Autodesk Fusion 360 part; units mm, degrees
(part 3 of 3)
  spline S37 degree 5 poles (-0.7155, 73.9902) (-0.7207, 73.9804) (-0.7312, 73.9608) (-0.7469, 73.9314) (-0.7676, 73.8922) (-0.7933, 73.8432) (-0.8188, 73.7941) (-0.844, 73.7449) (-0.8689, 73.6957) (-0.8936, 73.6465) (-0.9181, 73.5972) (-0.9422, 73.5478) (-0.9662, 73.4985) (-0.9898, 73.449) (-1.0133, 73.3995) (-1.0364, 73.35) (-1.0593, 73.3005) (-1.0819, 73.2509) (-1.1043, 73.2012) (-1.1264, 73.1515) (-1.1482, 73.1018) (-1.1697, 73.052) (-1.191, 73.0022) (-1.212, 72.9523) (-1.2327, 72.9025) (-1.2532, 72.8525) (-1.2733, 72.8026) (-1.2932, 72.7526) (-1.3128, 72.7025) (-1.3321, 72.6525) (-1.351, 72.6024) (-1.3697, 72.5522) (-1.3881, 72.502) (-1.4062, 72.4518) (-1.424, 72.4016) (-1.4415, 72.3513) (-1.4587, 72.301) (-1.4756, 72.2507) (-1.4921, 72.2004) (-1.5083, 72.15) (-1.5242, 72.0996) (-1.5398, 72.0491) (-1.555, 71.9987) (-1.5699, 71.9482) (-1.5844, 71.8977) (-1.5986, 71.8472) (-1.6124, 71.7966) (-1.6259, 71.7461) (-1.6391, 71.6955) (-1.6518, 71.6449) (-1.6642, 71.5943) (-1.6762, 71.5436) (-1.6877, 71.493) (-1.6988, 71.4423) (-1.7095, 71.3916) (-1.7198, 71.341) (-1.7297, 71.2903) (-1.7393, 71.2396) (-1.7484, 71.1889) (-1.7571, 71.1381) (-1.7652, 71.0874) (-1.7727, 71.0367) (-1.7795, 70.986) (-1.7856, 70.9353) (-1.7911, 70.8846) (-1.7962, 70.8339) (-1.801, 70.7832) (-1.8054, 70.7326) (-1.8093, 70.6819) (-1.8123, 70.6313) (-1.814, 70.5808) (-1.8137, 70.5404) (-1.8124, 70.5101) (-1.8111, 70.4899) (-1.8102, 70.4799) knots -1 -1 -1 -1 -1 -1 -0.98571429 -0.97142857 -0.95714286 -0.94285714 -0.92857143 -0.91428571 -0.9 -0.88571429 -0.87142857 -0.85714286 -0.84285714 -0.82857143 -0.81428571 -0.8 -0.78571429 -0.77142857 -0.75714286 -0.74285714 -0.72857143 -0.71428571 -0.7 -0.68571429 -0.67142857 -0.65714286 -0.64285714 -0.62857143 -0.61428571 -0.6 -0.58571429 -0.57142857 -0.55714286 -0.54285714 -0.52857143 -0.51428571 -0.5 -0.48571429 -0.47142857 -0.45714286 -0.44285714 -0.42857143 -0.41428571 -0.4 -0.38571429 -0.37142857 -0.35714286 -0.34285714 -0.32857143 -0.31428571 -0.3 -0.28571429 -0.27142857 -0.25714286 -0.24285714 -0.22857143 -0.21428571 -0.2 -0.18571429 -0.17142857 -0.15714286 -0.14285714 -0.12857143 -0.11428571 -0.1 -0.08571429 -0.07142857 -0.05714286 -0.04285714 -0.02857143 -0.01428571 0 0 0 0 0 0
  line L37 (-1.8102, 70.4799) -> (-1.8082, 70.4535)
  arc A75 (-2.6806, 69.3818) -> (-1.8082, 70.4535) centre (-2.805, 70.3741) ccw
  arc A76 (-2.6806, 69.3818) -> (-2.9448, 69.347) centre (0, 48) ccw
  arc A77 (-4.0649, 70.1564) -> (-2.9448, 69.347) centre (-3.0814, 70.3377) ccw
  line L38 (-4.0649, 70.1564) -> (-4.0696, 70.1824)
  spline S38 degree 5 poles (-4.0696, 70.1824) (-4.0715, 70.1923) (-4.0754, 70.2122) (-4.082, 70.2417) (-4.0922, 70.2808) (-4.1068, 70.3292) (-4.1229, 70.3773) (-4.1398, 70.4252) (-4.1571, 70.473) (-4.1748, 70.5207) (-4.1929, 70.5684) (-4.2113, 70.6159) (-4.2304, 70.6633) (-4.25, 70.7106) (-4.2704, 70.7576) (-4.2914, 70.8045) (-4.3129, 70.8512) (-4.3348, 70.8979) (-4.3572, 70.9444) (-4.3799, 70.9908) (-4.4029, 71.037) (-4.4264, 71.0832) (-4.4502, 71.1293) (-4.4745, 71.1752) (-4.4992, 71.221) (-4.5242, 71.2667) (-4.5496, 71.3123) (-4.5754, 71.3578) (-4.6015, 71.4031) (-4.628, 71.4484) (-4.6548, 71.4935) (-4.6819, 71.5385) (-4.7093, 71.5834) (-4.7371, 71.6282) (-4.7651, 71.6729) (-4.7935, 71.7175) (-4.8223, 71.7619) (-4.8513, 71.8063) (-4.8806, 71.8505) (-4.9102, 71.8947) (-4.9401, 71.9387) (-4.9703, 71.9826) (-5.0007, 72.0264) (-5.0315, 72.0701) (-5.0625, 72.1137) (-5.0939, 72.1572) (-5.1255, 72.2006) (-5.1573, 72.2438) (-5.1895, 72.287) (-5.2218, 72.33) (-5.2545, 72.373) (-5.2874, 72.4158) (-5.3206, 72.4585) (-5.3541, 72.5011) (-5.3878, 72.5436) (-5.4217, 72.586) (-5.4559, 72.6283) (-5.4903, 72.6705) (-5.525, 72.7125) (-5.56, 72.7545) (-5.5952, 72.7963) (-5.6306, 72.8381) (-5.6662, 72.8797) (-5.7021, 72.9212) (-5.7383, 72.9626) (-5.7746, 73.0039) (-5.8112, 73.0451) (-5.8481, 73.0861) (-5.8851, 73.1271) (-5.9224, 73.1679) (-5.9599, 73.2086) (-5.9901, 73.2411) (-6.0128, 73.2655) (-6.0281, 73.2816) (-6.0357, 73.2897) knots 0 0 0 0 0 0 0.01428571 0.02857143 0.04285714 0.05714286 0.07142857 0.08571429 0.1 0.11428571 0.12857143 0.14285714 0.15714286 0.17142857 0.18571429 0.2 0.21428571 0.22857143 0.24285714 0.25714286 0.27142857 0.28571429 0.3 0.31428571 0.32857143 0.34285714 0.35714286 0.37142857 0.38571429 0.4 0.41428571 0.42857143 0.44285714 0.45714286 0.47142857 0.48571429 0.5 0.51428571 0.52857143 0.54285714 0.55714286 0.57142857 0.58571429 0.6 0.61428571 0.62857143 0.64285714 0.65714286 0.67142857 0.68571429 0.7 0.71428571 0.72857143 0.74285714 0.75714286 0.77142857 0.78571429 0.8 0.81428571 0.82857143 0.84285714 0.85714286 0.87142857 0.88571429 0.9 0.91428571 0.92857143 0.94285714 0.95714286 0.97142857 0.98571429 1 1 1 1 1 1
  arc A78 (-6.0357, 73.2897) -> (-7.4178, 72.9194) centre (0, 48) ccw
  spline S39 degree 5 poles (-7.4178, 72.9194) (-7.4204, 72.9086) (-7.4255, 72.8869) (-7.433, 72.8545) (-7.4429, 72.8113) (-7.455, 72.7573) (-7.4669, 72.7032) (-7.4785, 72.6492) (-7.4899, 72.5953) (-7.501, 72.5413) (-7.5118, 72.4874) (-7.5224, 72.4335) (-7.5327, 72.3796) (-7.5428, 72.3257) (-7.5526, 72.2718) (-7.5622, 72.218) (-7.5714, 72.1642) (-7.5805, 72.1104) (-7.5892, 72.0567) (-7.5977, 72.003) (-7.6059, 71.9493) (-7.6138, 71.8956) (-7.6215, 71.842) (-7.6289, 71.7884) (-7.636, 71.7349) (-7.6428, 71.6814) (-7.6493, 71.6279) (-7.6556, 71.5744) (-7.6615, 71.521) (-7.6672, 71.4677) (-7.6726, 71.4144) (-7.6777, 71.3611) (-7.6824, 71.3079) (-7.6869, 71.2547) (-7.6911, 71.2016) (-7.695, 71.1485) (-7.6986, 71.0955) (-7.7018, 71.0425) (-7.7048, 70.9896) (-7.7074, 70.9367) (-7.7097, 70.8839) (-7.7117, 70.8312) (-7.7133, 70.7785) (-7.7146, 70.7259) (-7.7156, 70.6733) (-7.7162, 70.6209) (-7.7165, 70.5685) (-7.7165, 70.5161) (-7.7161, 70.4639) (-7.7153, 70.4117) (-7.7141, 70.3596) (-7.7126, 70.3076) (-7.7106, 70.2557) (-7.7083, 70.2039) (-7.7055, 70.1521) (-7.7023, 70.1005) (-7.6988, 70.049) (-7.6948, 69.9975) (-7.6906, 69.9462) (-7.6858, 69.895) (-7.6805, 69.8439) (-7.6746, 69.7929) (-7.6681, 69.7422) (-7.6609, 69.6916) (-7.6531, 69.6412) (-7.6449, 69.591) (-7.6363, 69.5408) (-7.6275, 69.4907) (-7.6182, 69.4408) (-7.608, 69.3911) (-7.5965, 69.3419) (-7.5858, 69.3029) (-7.5767, 69.274) (-7.5702, 69.2549) (-7.5668, 69.2453) knots -1 -1 -1 -1 -1 -1 -0.98571429 -0.97142857 -0.95714286 -0.94285714 -0.92857143 -0.91428571 -0.9 -0.88571429 -0.87142857 -0.85714286 -0.84285714 -0.82857143 -0.81428571 -0.8 -0.78571429 -0.77142857 -0.75714286 -0.74285714 -0.72857143 -0.71428571 -0.7 -0.68571429 -0.67142857 -0.65714286 -0.64285714 -0.62857143 -0.61428571 -0.6 -0.58571429 -0.57142857 -0.55714286 -0.54285714 -0.52857143 -0.51428571 -0.5 -0.48571429 -0.47142857 -0.45714286 -0.44285714 -0.42857143 -0.41428571 -0.4 -0.38571429 -0.37142857 -0.35714286 -0.34285714 -0.32857143 -0.31428571 -0.3 -0.28571429 -0.27142857 -0.25714286 -0.24285714 -0.22857143 -0.21428571 -0.2 -0.18571429 -0.17142857 -0.15714286 -0.14285714 -0.12857143 -0.11428571 -0.1 -0.08571429 -0.07142857 -0.05714286 -0.04285714 -0.02857143 -0.01428571 0 0 0 0 0 0
  line L39 (-7.5668, 69.2453) -> (-7.5579, 69.2205)
  arc A79 (-8.1233, 67.9595) -> (-7.5579, 69.2205) centre (-8.5002, 68.8857) ccw
  arc A80 (-8.1233, 67.9595) -> (-8.3695, 67.8575) centre (0, 48) ccw
  arc A81 (-9.6609, 68.3494) -> (-8.3695, 67.8575) centre (-8.7578, 68.779) ccw
  line L40 (-9.6609, 68.3494) -> (-9.6722, 68.3732)
  spline S40 degree 5 poles (-9.6722, 68.3732) (-9.6765, 68.3824) (-9.6855, 68.4005) (-9.6995, 68.4274) (-9.7194, 68.4625) (-9.7461, 68.5055) (-9.7741, 68.5478) (-9.8028, 68.5897) (-9.8319, 68.6313) (-9.8614, 68.6728) (-9.8911, 68.7142) (-9.9213, 68.7554) (-9.9519, 68.7962) (-9.9832, 68.8367) (-10.015, 68.8769) (-10.0474, 68.9168) (-10.0803, 68.9563) (-10.1135, 68.9957) (-10.1471, 69.0348) (-10.1811, 69.0738) (-10.2153, 69.1125) (-10.2499, 69.1511) (-10.2849, 69.1894) (-10.3202, 69.2275) (-10.3559, 69.2653) (-10.3919, 69.303) (-10.4283, 69.3404) (-10.4649, 69.3777) (-10.5019, 69.4147) (-10.5392, 69.4516) (-10.5767, 69.4882) (-10.6146, 69.5247) (-10.6527, 69.561) (-10.6911, 69.5971) (-10.7298, 69.633) (-10.7687, 69.6687) (-10.808, 69.7042) (-10.8475, 69.7395) (-10.8873, 69.7747) (-10.9273, 69.8096) (-10.9675, 69.8444) (-11.0081, 69.879) (-11.0488, 69.9135) (-11.0899, 69.9477) (-11.1311, 69.9818) (-11.1726, 70.0157) (-11.2144, 70.0494) (-11.2564, 70.0829) (-11.2986, 70.1163) (-11.341, 70.1495) (-11.3837, 70.1825) (-11.4265, 70.2154) (-11.4697, 70.248) (-11.513, 70.2805) (-11.5565, 70.3129) (-11.6003, 70.345) (-11.6443, 70.377) (-11.6885, 70.4088) (-11.7329, 70.4405) (-11.7775, 70.472) (-11.8223, 70.5033) (-11.8673, 70.5344) (-11.9125, 70.5654) (-11.9579, 70.5962) (-12.0035, 70.6268) (-12.0493, 70.6573) (-12.0954, 70.6876) (-12.1416, 70.7177) (-12.188, 70.7477) (-12.2345, 70.7775) (-12.2813, 70.8071) (-12.3189, 70.8307) (-12.3471, 70.8483) (-12.366, 70.86) (-12.3755, 70.8659) knots 0 0 0 0 0 0 0.01428571 0.02857143 0.04285714 0.05714286 0.07142857 0.08571429 0.1 0.11428571 0.12857143 0.14285714 0.15714286 0.17142857 0.18571429 0.2 0.21428571 0.22857143 0.24285714 0.25714286 0.27142857 0.28571429 0.3 0.31428571 0.32857143 0.34285714 0.35714286 0.37142857 0.38571429 0.4 0.41428571 0.42857143 0.44285714 0.45714286 0.47142857 0.48571429 0.5 0.51428571 0.52857143 0.54285714 0.55714286 0.57142857 0.58571429 0.6 0.61428571 0.62857143 0.64285714 0.65714286 0.67142857 0.68571429 0.7 0.71428571 0.72857143 0.74285714 0.75714286 0.77142857 0.78571429 0.8 0.81428571 0.82857143 0.84285714 0.85714286 0.87142857 0.88571429 0.9 0.91428571 0.92857143 0.94285714 0.95714286 0.97142857 0.98571429 1 1 1 1 1 1
  arc A82 (-12.3755, 70.8659) -> (-13.6147, 70.1504) centre (0, 48) ccw
  spline S41 degree 5 poles (-13.6147, 70.1504) (-13.6143, 70.1393) (-13.6137, 70.1171) (-13.6125, 70.0838) (-13.6109, 70.0395) (-13.6086, 69.9842) (-13.6061, 69.9289) (-13.6034, 69.8738) (-13.6004, 69.8187) (-13.5971, 69.7637) (-13.5936, 69.7088) (-13.5899, 69.654) (-13.586, 69.5992) (-13.5817, 69.5446) (-13.5773, 69.49) (-13.5726, 69.4356) (-13.5676, 69.3812) (-13.5624, 69.3269) (-13.5569, 69.2727) (-13.5512, 69.2187) (-13.5453, 69.1647) (-13.539, 69.1108) (-13.5325, 69.057) (-13.5258, 69.0034) (-13.5188, 68.9498) (-13.5115, 68.8963) (-13.504, 68.843) (-13.4962, 68.7898) (-13.4882, 68.7366) (-13.4798, 68.6836) (-13.4712, 68.6307) (-13.4623, 68.578) (-13.4532, 68.5253) (-13.4438, 68.4728) (-13.4341, 68.4204) (-13.4241, 68.3681) (-13.4138, 68.316) (-13.4032, 68.264) (-13.3924, 68.2121) (-13.3812, 68.1603) (-13.3698, 68.1087) (-13.3581, 68.0573) (-13.346, 68.006) (-13.3337, 67.9548) (-13.321, 67.9038) (-13.308, 67.853) (-13.2947, 67.8023) (-13.2811, 67.7517) (-13.2672, 67.7014) (-13.253, 67.6512) (-13.2384, 67.6011) (-13.2234, 67.5513) (-13.2081, 67.5017) (-13.1924, 67.4522) (-13.1763, 67.403) (-13.1599, 67.354) (-13.1431, 67.3051) (-13.126, 67.2564) (-13.1086, 67.2079) (-13.0908, 67.1597) (-13.0724, 67.1117) (-13.0536, 67.064) (-13.0341, 67.0167) (-13.014, 66.9697) (-12.9935, 66.9231) (-12.9725, 66.8766) (-12.9513, 66.8304) (-12.9298, 66.7843) (-12.9079, 66.7385) (-12.8852, 66.6931) (-12.8613, 66.6485) (-12.8409, 66.6137) (-12.8246, 66.5881) (-12.8134, 66.5713) (-12.8076, 66.563) knots -1 -1 -1 -1 -1 -1 -0.98571429 -0.97142857 -0.95714286 -0.94285714 -0.92857143 -0.91428571 -0.9 -0.88571429 -0.87142857 -0.85714286 -0.84285714 -0.82857143 -0.81428571 -0.8 -0.78571429 -0.77142857 -0.75714286 -0.74285714 -0.72857143 -0.71428571 -0.7 -0.68571429 -0.67142857 -0.65714286 -0.64285714 -0.62857143 -0.61428571 -0.6 -0.58571429 -0.57142857 -0.55714286 -0.54285714 -0.52857143 -0.51428571 -0.5 -0.48571429 -0.47142857 -0.45714286 -0.44285714 -0.42857143 -0.41428571 -0.4 -0.38571429 -0.37142857 -0.35714286 -0.34285714 -0.32857143 -0.31428571 -0.3 -0.28571429 -0.27142857 -0.25714286 -0.24285714 -0.22857143 -0.21428571 -0.2 -0.18571429 -0.17142857 -0.15714286 -0.14285714 -0.12857143 -0.11428571 -0.1 -0.08571429 -0.07142857 -0.05714286 -0.04285714 -0.02857143 -0.01428571 0 0 0 0 0 0
  line L41 (-12.8076, 66.563) -> (-12.7927, 66.5413)
  arc A83 (-13.0124, 65.1769) -> (-12.7927, 66.5413) centre (-13.6162, 65.974) ccw
  arc A84 (-13.0124, 65.1769) -> (-13.2238, 65.0147) centre (0, 48) ccw
  arc A85 (-14.5985, 65.1556) -> (-13.2238, 65.0147) centre (-13.8374, 65.8043) ccw
  line L42 (-14.5985, 65.1556) -> (-14.6156, 65.1757)
  spline S42 degree 5 poles (-14.6156, 65.1757) (-14.6222, 65.1834) (-14.6355, 65.1986) (-14.656, 65.2209) (-14.6843, 65.2497) (-14.7212, 65.2843) (-14.7592, 65.3179) (-14.7977, 65.3509) (-14.8367, 65.3836) (-14.8759, 65.4161) (-14.9153, 65.4484) (-14.9551, 65.4803) (-14.9953, 65.5119) (-15.0359, 65.5429) (-15.0771, 65.5735) (-15.1187, 65.6036) (-15.1607, 65.6333) (-15.203, 65.6627) (-15.2456, 65.6918) (-15.2885, 65.7206) (-15.3316, 65.7492) (-15.375, 65.7775) (-15.4187, 65.8054) (-15.4626, 65.8331) (-15.5069, 65.8604) (-15.5514, 65.8875) (-15.5963, 65.9142) (-15.6413, 65.9407) (-15.6866, 65.9669) (-15.7321, 65.9929) (-15.7779, 66.0186) (-15.8239, 66.044) (-15.8701, 66.0692) (-15.9165, 66.0941) (-15.9632, 66.1188) (-16.0101, 66.1432) (-16.0572, 66.1673) (-16.1045, 66.1912) (-16.152, 66.2149) (-16.1997, 66.2383) (-16.2476, 66.2615) (-16.2957, 66.2844) (-16.344, 66.3071) (-16.3925, 66.3296) (-16.4412, 66.3518) (-16.49, 66.3738) (-16.5391, 66.3956) (-16.5883, 66.4171) (-16.6377, 66.4384) (-16.6873, 66.4595) (-16.737, 66.4804) (-16.787, 66.501) (-16.8371, 66.5214) (-16.8873, 66.5416) (-16.9377, 66.5615) (-16.9883, 66.5813) (-17.0391, 66.6008) (-17.09, 66.6201) (-17.1411, 66.6392) (-17.1923, 66.658) (-17.2437, 66.6767) (-17.2953, 66.6951) (-17.3469, 66.7133) (-17.3988, 66.7313) (-17.4508, 66.7491) (-17.5029, 66.7667) (-17.5552, 66.784) (-17.6076, 66.8012) (-17.6602, 66.8181) (-17.7129, 66.8348) (-17.7658, 66.8514) (-17.8081, 66.8644) (-17.84, 66.8741) (-17.8613, 66.8805) (-17.8719, 66.8837) knots 0 0 0 0 0 0 0.01428571 0.02857143 0.04285714 0.05714286 0.07142857 0.08571429 0.1 0.11428571 0.12857143 0.14285714 0.15714286 0.17142857 0.18571429 0.2 0.21428571 0.22857143 0.24285714 0.25714286 0.27142857 0.28571429 0.3 0.31428571 0.32857143 0.34285714 0.35714286 0.37142857 0.38571429 0.4 0.41428571 0.42857143 0.44285714 0.45714286 0.47142857 0.48571429 0.5 0.51428571 0.52857143 0.54285714 0.55714286 0.57142857 0.58571429 0.6 0.61428571 0.62857143 0.64285714 0.65714286 0.67142857 0.68571429 0.7 0.71428571 0.72857143 0.74285714 0.75714286 0.77142857 0.78571429 0.8 0.81428571 0.82857143 0.84285714 0.85714286 0.87142857 0.88571429 0.9 0.91428571 0.92857143 0.94285714 0.95714286 0.97142857 0.98571429 1 1 1 1 1 1
  arc A86 (-17.8719, 66.8837) -> (-18.8837, 65.8719) centre (0, 48) ccw
  spline S43 degree 5 poles (-18.8837, 65.8719) (-18.8805, 65.8613) (-18.8741, 65.84) (-18.8644, 65.8081) (-18.8514, 65.7658) (-18.8348, 65.7129) (-18.8181, 65.6602) (-18.8012, 65.6076) (-18.784, 65.5552) (-18.7667, 65.5029) (-18.7491, 65.4508) (-18.7313, 65.3988) (-18.7133, 65.3469) (-18.6951, 65.2953) (-18.6767, 65.2437) (-18.658, 65.1923) (-18.6392, 65.1411) (-18.6201, 65.09) (-18.6008, 65.0391) (-18.5813, 64.9883) (-18.5615, 64.9377) (-18.5416, 64.8873) (-18.5214, 64.8371) (-18.501, 64.787) (-18.4804, 64.737) (-18.4595, 64.6873) (-18.4384, 64.6377) (-18.4171, 64.5883) (-18.3956, 64.5391) (-18.3738, 64.49) (-18.3518, 64.4412) (-18.3296, 64.3925) (-18.3071, 64.344) (-18.2844, 64.2957) (-18.2615, 64.2476) (-18.2383, 64.1997) (-18.2149, 64.152) (-18.1912, 64.1045) (-18.1673, 64.0572) (-18.1432, 64.0101) (-18.1188, 63.9632) (-18.0941, 63.9165) (-18.0692, 63.8701) (-18.044, 63.8239) (-18.0186, 63.7779) (-17.9929, 63.7321) (-17.9669, 63.6866) (-17.9407, 63.6413) (-17.9142, 63.5963) (-17.8875, 63.5514) (-17.8604, 63.5069) (-17.8331, 63.4626) (-17.8054, 63.4187) (-17.7775, 63.375) (-17.7492, 63.3316) (-17.7206, 63.2885) (-17.6918, 63.2456) (-17.6627, 63.203) (-17.6333, 63.1607) (-17.6036, 63.1187) (-17.5735, 63.0771) (-17.5429, 63.0359) (-17.5119, 62.9953) (-17.4803, 62.9551) (-17.4484, 62.9153) (-17.4161, 62.8759) (-17.3836, 62.8367) (-17.3509, 62.7977) (-17.3179, 62.7592) (-17.2843, 62.7212) (-17.2497, 62.6843) (-17.2209, 62.656) (-17.1986, 62.6355) (-17.1834, 62.6222) (-17.1757, 62.6156) knots -1 -1 -1 -1 -1 -1 -0.98571429 -0.97142857 -0.95714286 -0.94285714 -0.92857143 -0.91428571 -0.9 -0.88571429 -0.87142857 -0.85714286 -0.84285714 -0.82857143 -0.81428571 -0.8 -0.78571429 -0.77142857 -0.75714286 -0.74285714 -0.72857143 -0.71428571 -0.7 -0.68571429 -0.67142857 -0.65714286 -0.64285714 -0.62857143 -0.61428571 -0.6 -0.58571429 -0.57142857 -0.55714286 -0.54285714 -0.52857143 -0.51428571 -0.5 -0.48571429 -0.47142857 -0.45714286 -0.44285714 -0.42857143 -0.41428571 -0.4 -0.38571429 -0.37142857 -0.35714286 -0.34285714 -0.32857143 -0.31428571 -0.3 -0.28571429 -0.27142857 -0.25714286 -0.24285714 -0.22857143 -0.21428571 -0.2 -0.18571429 -0.17142857 -0.15714286 -0.14285714 -0.12857143 -0.11428571 -0.1 -0.08571429 -0.07142857 -0.05714286 -0.04285714 -0.02857143 -0.01428571 0 0 0 0 0 0
  line L43 (-17.1757, 62.6156) -> (-17.1556, 62.5985)
  arc A87 (-17.0147, 61.2238) -> (-17.1556, 62.5985) centre (-17.8043, 61.8374) ccw
  arc A88 (-17.0147, 61.2238) -> (-17.1769, 61.0124) centre (0, 48) ccw
  arc A89 (-18.5413, 60.7927) -> (-17.1769, 61.0124) centre (-17.974, 61.6162) ccw
  line L44 (-18.5413, 60.7927) -> (-18.563, 60.8076)
  spline S44 degree 5 poles (-18.563, 60.8076) (-18.5713, 60.8134) (-18.5881, 60.8246) (-18.6137, 60.8409) (-18.6485, 60.8613) (-18.6931, 60.8852) (-18.7385, 60.9079) (-18.7843, 60.9298) (-18.8304, 60.9513) (-18.8766, 60.9725) (-18.9231, 60.9935) (-18.9697, 61.014) (-19.0167, 61.0341) (-19.064, 61.0536) (-19.1117, 61.0724) (-19.1597, 61.0908) (-19.2079, 61.1086) (-19.2564, 61.126) (-19.3051, 61.1431) (-19.354, 61.1599) (-19.403, 61.1763) (-19.4522, 61.1924) (-19.5017, 61.2081) (-19.5513, 61.2234) (-19.6011, 61.2384) (-19.6512, 61.253) (-19.7014, 61.2672) (-19.7517, 61.2811) (-19.8023, 61.2947) (-19.853, 61.308) (-19.9038, 61.321) (-19.9548, 61.3337) (-20.006, 61.346) (-20.0573, 61.3581) (-20.1087, 61.3698) (-20.1603, 61.3812) (-20.2121, 61.3924) (-20.264, 61.4032) (-20.316, 61.4138) (-20.3681, 61.4241) (-20.4204, 61.4341) (-20.4728, 61.4438) (-20.5253, 61.4532) (-20.578, 61.4623) (-20.6307, 61.4712) (-20.6836, 61.4798) (-20.7366, 61.4882) (-20.7898, 61.4962) (-20.843, 61.504) (-20.8963, 61.5115) (-20.9498, 61.5188) (-21.0034, 61.5258) (-21.057, 61.5325) (-21.1108, 61.539) (-21.1647, 61.5453) (-21.2187, 61.5512) (-21.2727, 61.5569) (-21.3269, 61.5624) (-21.3812, 61.5676) (-21.4356, 61.5726) (-21.49, 61.5773) (-21.5446, 61.5817) (-21.5992, 61.586) (-21.654, 61.5899) (-21.7088, 61.5936) (-21.7637, 61.5971) (-21.8187, 61.6004) (-21.8738, 61.6034) (-21.9289, 61.6061) (-21.9842, 61.6086) (-22.0395, 61.6109) (-22.0838, 61.6125) (-22.1171, 61.6137) (-22.1393, 61.6143) (-22.1504, 61.6147) knots 0 0 0 0 0 0 0.01428571 0.02857143 0.04285714 0.05714286 0.07142857 0.08571429 0.1 0.11428571 0.12857143 0.14285714 0.15714286 0.17142857 0.18571429 0.2 0.21428571 0.22857143 0.24285714 0.25714286 0.27142857 0.28571429 0.3 0.31428571 0.32857143 0.34285714 0.35714286 0.37142857 0.38571429 0.4 0.41428571 0.42857143 0.44285714 0.45714286 0.47142857 0.48571429 0.5 0.51428571 0.52857143 0.54285714 0.55714286 0.57142857 0.58571429 0.6 0.61428571 0.62857143 0.64285714 0.65714286 0.67142857 0.68571429 0.7 0.71428571 0.72857143 0.74285714 0.75714286 0.77142857 0.78571429 0.8 0.81428571 0.82857143 0.84285714 0.85714286 0.87142857 0.88571429 0.9 0.91428571 0.92857143 0.94285714 0.95714286 0.97142857 0.98571429 1 1 1 1 1 1
  arc A90 (-22.1504, 61.6147) -> (-22.8659, 60.3755) centre (0, 48) ccw
  spline S45 degree 5 poles (-22.8659, 60.3755) (-22.86, 60.366) (-22.8483, 60.3471) (-22.8307, 60.3189) (-22.8071, 60.2813) (-22.7775, 60.2345) (-22.7477, 60.188) (-22.7177, 60.1416) (-22.6876, 60.0954) (-22.6573, 60.0493) (-22.6268, 60.0035) (-22.5962, 59.9579) (-22.5654, 59.9125) (-22.5344, 59.8673) (-22.5033, 59.8223) (-22.472, 59.7775) (-22.4405, 59.7329) (-22.4088, 59.6885) (-22.377, 59.6443) (-22.345, 59.6003) (-22.3129, 59.5565) (-22.2805, 59.513) (-22.248, 59.4697) (-22.2154, 59.4265) (-22.1825, 59.3837) (-22.1495, 59.341) (-22.1163, 59.2986) (-22.0829, 59.2564) (-22.0494, 59.2144) (-22.0157, 59.1726) (-21.9818, 59.1311) (-21.9477, 59.0899) (-21.9135, 59.0488) (-21.879, 59.0081) (-21.8444, 58.9675) (-21.8096, 58.9273) (-21.7747, 58.8873) (-21.7395, 58.8475) (-21.7042, 58.808) (-21.6687, 58.7687) (-21.633, 58.7298) (-21.5971, 58.6911) (-21.561, 58.6527) (-21.5247, 58.6146) (-21.4882, 58.5767) (-21.4516, 58.5392) (-21.4147, 58.5019) (-21.3777, 58.4649) (-21.3404, 58.4283) (-21.303, 58.3919) (-21.2653, 58.3559) (-21.2275, 58.3202) (-21.1894, 58.2849) (-21.1511, 58.2499) (-21.1125, 58.2153) (-21.0738, 58.1811) (-21.0348, 58.1471) (-20.9957, 58.1135) (-20.9563, 58.0803) (-20.9168, 58.0474) (-20.8769, 58.015) (-20.8367, 57.9832) (-20.7962, 57.9519) (-20.7554, 57.9213) (-20.7142, 57.8911) (-20.6728, 57.8614) (-20.6313, 57.8319) (-20.5897, 57.8028) (-20.5478, 57.7741) (-20.5055, 57.7461) (-20.4625, 57.7194) (-20.4274, 57.6995) (-20.4005, 57.6855) (-20.3824, 57.6765) (-20.3732, 57.6722) knots -1 -1 -1 -1 -1 -1 -0.98571429 -0.97142857 -0.95714286 -0.94285714 -0.92857143 -0.91428571 -0.9 -0.88571429 -0.87142857 -0.85714286 -0.84285714 -0.82857143 -0.81428571 -0.8 -0.78571429 -0.77142857 -0.75714286 -0.74285714 -0.72857143 -0.71428571 -0.7 -0.68571429 -0.67142857 -0.65714286 -0.64285714 -0.62857143 -0.61428571 -0.6 -0.58571429 -0.57142857 -0.55714286 -0.54285714 -0.52857143 -0.51428571 -0.5 -0.48571429 -0.47142857 -0.45714286 -0.44285714 -0.42857143 -0.41428571 -0.4 -0.38571429 -0.37142857 -0.35714286 -0.34285714 -0.32857143 -0.31428571 -0.3 -0.28571429 -0.27142857 -0.25714286 -0.24285714 -0.22857143 -0.21428571 -0.2 -0.18571429 -0.17142857 -0.15714286 -0.14285714 -0.12857143 -0.11428571 -0.1 -0.08571429 -0.07142857 -0.05714286 -0.04285714 -0.02857143 -0.01428571 0 0 0 0 0 0
  line L45 (-20.3732, 57.6722) -> (-20.3494, 57.6609)
  arc A91 (-19.8575, 56.3695) -> (-20.3494, 57.6609) centre (-20.779, 56.7578) ccw
  arc A92 (-19.8575, 56.3695) -> (-19.9595, 56.1233) centre (0, 48) ccw
  arc A93 (-21.2205, 55.5579) -> (-19.9595, 56.1233) centre (-20.8857, 56.5002) ccw
  line L46 (-21.2205, 55.5579) -> (-21.2453, 55.5668)
  spline S46 degree 5 poles (-21.2453, 55.5668) (-21.2549, 55.5702) (-21.274, 55.5767) (-21.3029, 55.5858) (-21.3419, 55.5965) (-21.3911, 55.608) (-21.4408, 55.6182) (-21.4907, 55.6275) (-21.5408, 55.6363) (-21.591, 55.6449) (-21.6412, 55.6531) (-21.6916, 55.6609) (-21.7422, 55.6681) (-21.7929, 55.6746) (-21.8439, 55.6805) (-21.895, 55.6858) (-21.9462, 55.6906) (-21.9975, 55.6948) (-22.049, 55.6988) (-22.1005, 55.7023) (-22.1521, 55.7055) (-22.2039, 55.7083) (-22.2557, 55.7106) (-22.3076, 55.7126) (-22.3596, 55.7141) (-22.4117, 55.7153) (-22.4639, 55.7161) (-22.5161, 55.7165) (-22.5685, 55.7165) (-22.6209, 55.7162) (-22.6733, 55.7156) (-22.7259, 55.7146) (-22.7785, 55.7133) (-22.8312, 55.7117) (-22.8839, 55.7097) (-22.9367, 55.7074) (-22.9896, 55.7048) (-23.0425, 55.7018) (-23.0955, 55.6986) (-23.1485, 55.695) (-23.2016, 55.6911) (-23.2547, 55.6869) (-23.3079, 55.6824) (-23.3611, 55.6777) (-23.4144, 55.6726) (-23.4677, 55.6672) (-23.521, 55.6615) (-23.5744, 55.6556) (-23.6279, 55.6493) (-23.6814, 55.6428) (-23.7349, 55.636) (-23.7884, 55.6289) (-23.842, 55.6215) (-23.8956, 55.6138) (-23.9493, 55.6059) (-24.003, 55.5977) (-24.0567, 55.5892) (-24.1104, 55.5805) (-24.1642, 55.5714) (-24.218, 55.5622) (-24.2718, 55.5526) (-24.3257, 55.5428) (-24.3796, 55.5327) (-24.4335, 55.5224) (-24.4874, 55.5118) (-24.5413, 55.501) (-24.5953, 55.4899) (-24.6492, 55.4785) (-24.7032, 55.4669) (-24.7573, 55.455) (-24.8113, 55.4429) (-24.8545, 55.433) (-24.8869, 55.4255) (-24.9086, 55.4204) (-24.9194, 55.4178) knots 0 0 0 0 0 0 0.01428571 0.02857143 0.04285714 0.05714286 0.07142857 0.08571429 0.1 0.11428571 0.12857143 0.14285714 0.15714286 0.17142857 0.18571429 0.2 0.21428571 0.22857143 0.24285714 0.25714286 0.27142857 0.28571429 0.3 0.31428571 0.32857143 0.34285714 0.35714286 0.37142857 0.38571429 0.4 0.41428571 0.42857143 0.44285714 0.45714286 0.47142857 0.48571429 0.5 0.51428571 0.52857143 0.54285714 0.55714286 0.57142857 0.58571429 0.6 0.61428571 0.62857143 0.64285714 0.65714286 0.67142857 0.68571429 0.7 0.71428571 0.72857143 0.74285714 0.75714286 0.77142857 0.78571429 0.8 0.81428571 0.82857143 0.84285714 0.85714286 0.87142857 0.88571429 0.9 0.91428571 0.92857143 0.94285714 0.95714286 0.97142857 0.98571429 1 1 1 1 1 1
  arc A94 (-24.9194, 55.4178) -> (-25.2897, 54.0357) centre (0, 48) ccw
  spline S47 degree 5 poles (-25.2897, 54.0357) (-25.2816, 54.0281) (-25.2655, 54.0128) (-25.2411, 53.9901) (-25.2086, 53.9599) (-25.1679, 53.9224) (-25.1271, 53.8851) (-25.0861, 53.8481) (-25.0451, 53.8112) (-25.0039, 53.7746) (-24.9626, 53.7383) (-24.9212, 53.7021) (-24.8797, 53.6662) (-24.8381, 53.6306) (-24.7963, 53.5952) (-24.7545, 53.56) (-24.7125, 53.525) (-24.6705, 53.4903) (-24.6283, 53.4559) (-24.586, 53.4217) (-24.5436, 53.3878) (-24.5011, 53.3541) (-24.4585, 53.3206) (-24.4158, 53.2874) (-24.373, 53.2545) (-24.33, 53.2218) (-24.287, 53.1895) (-24.2438, 53.1573) (-24.2006, 53.1255) (-24.1572, 53.0939) (-24.1137, 53.0625) (-24.0701, 53.0315) (-24.0264, 53.0007) (-23.9826, 52.9703) (-23.9387, 52.9401) (-23.8947, 52.9102) (-23.8505, 52.8806) (-23.8063, 52.8513) (-23.7619, 52.8223) (-23.7175, 52.7935) (-23.6729, 52.7651) (-23.6282, 52.7371) (-23.5834, 52.7093) (-23.5385, 52.6819) (-23.4935, 52.6548) (-23.4484, 52.628) (-23.4031, 52.6015) (-23.3578, 52.5754) (-23.3123, 52.5496) (-23.2667, 52.5242) (-23.221, 52.4992) (-23.1752, 52.4745) (-23.1293, 52.4502) (-23.0832, 52.4264) (-23.037, 52.4029) (-22.9908, 52.3799) (-22.9444, 52.3572) (-22.8979, 52.3348) (-22.8512, 52.3129) (-22.8045, 52.2914) (-22.7576, 52.2704) (-22.7106, 52.25) (-22.6633, 52.2304) (-22.6159, 52.2113) (-22.5684, 52.1929) (-22.5207, 52.1748) (-22.473, 52.1571) (-22.4252, 52.1398) (-22.3773, 52.1229) (-22.3292, 52.1068) (-22.2808, 52.0922) (-22.2417, 52.082) (-22.2122, 52.0754) (-22.1923, 52.0715) (-22.1824, 52.0696) knots -1 -1 -1 -1 -1 -1 -0.98571429 -0.97142857 -0.95714286 -0.94285714 -0.92857143 -0.91428571 -0.9 -0.88571429 -0.87142857 -0.85714286 -0.84285714 -0.82857143 -0.81428571 -0.8 -0.78571429 -0.77142857 -0.75714286 -0.74285714 -0.72857143 -0.71428571 -0.7 -0.68571429 -0.67142857 -0.65714286 -0.64285714 -0.62857143 -0.61428571 -0.6 -0.58571429 -0.57142857 -0.55714286 -0.54285714 -0.52857143 -0.51428571 -0.5 -0.48571429 -0.47142857 -0.45714286 -0.44285714 -0.42857143 -0.41428571 -0.4 -0.38571429 -0.37142857 -0.35714286 -0.34285714 -0.32857143 -0.31428571 -0.3 -0.28571429 -0.27142857 -0.25714286 -0.24285714 -0.22857143 -0.21428571 -0.2 -0.18571429 -0.17142857 -0.15714286 -0.14285714 -0.12857143 -0.11428571 -0.1 -0.08571429 -0.07142857 -0.05714286 -0.04285714 -0.02857143 -0.01428571 0 0 0 0 0 0
  line L47 (-22.1824, 52.0696) -> (-22.1564, 52.0649)
  arc A95 (-21.347, 50.9448) -> (-22.1564, 52.0649) centre (-22.3377, 51.0814) ccw
  circle A96 centre (0, 48) radius 6.35
  line L48 (2.6806, 26.6182) -> (-2.8127, 26.6352)
  constraint coincident A27.start A28.start
  constraint midpoint A24 L48.end
extrude "押し出し1'" add sketch "スケッチ1 (2)" against normal blind 12.7 separate body contours A24 A25 L12 S12 A26 S13 L13 A27 L48 makes body 3 in component "Rack"
delete_body "RemoveBody1" bodies 2 in component "Rack"
pattern_linear "R パターン1" count 21 spacing 6.2832 along (0.999995, -0.003091, 0) both ways of bodies 3 makes body 4 at (-63.681, -26.4296, 4.2333) makes body 5 at (-57.3979, -26.449, 4.2333) makes body 6 at (-51.1147, -26.4685, 4.2333) makes body 7 at (-44.8316, -26.4879, 4.2333) makes body 8 at (-38.5484, -26.5073, 4.2333) makes body 9 at (-32.2653, -26.5267, 4.2333) makes body 10 at (-25.9821, -26.5461, 4.2333) makes body 11 at (-19.6989, -26.5656, 4.2333) makes body 12 at (-13.4158, -26.585, 4.2333) makes body 13 at (-7.1326, -26.6044, 8.4667) makes body 14 at (5.4337, -26.6433, 4.2333) makes body 15 at (11.7168, -26.6627, 4.2333) makes body 16 at (18, -26.6821, 4.2333) makes body 17 at (24.2831, -26.7015, 4.2333) makes body 18 at (30.5663, -26.721, 4.2333) makes body 19 at (36.8494, -26.7404, 4.2333) makes body 20 at (43.1326, -26.7598, 4.2333) makes body 21 at (49.4158, -26.7792, 4.2333) makes body 22 at (55.6989, -26.7986, 4.2333) makes body 23 at (61.9821, -26.8181, 8.4667) in component "Rack"
sketch "スケッチ2 (2)" plane through (0, 0, 12.7) normal (0, 0, 1) x (-1, 0, 0) in component "Rack"
  line L0 (-1.8082, 25.5465) -> (-1.8102, 25.5201)
  spline S0 degree 5 poles (-1.8102, 25.5201) (-1.8111, 25.5101) (-1.8124, 25.4899) (-1.8137, 25.4596) (-1.814, 25.4192) (-1.8123, 25.3687) (-1.8093, 25.3181) (-1.8054, 25.2674) (-1.801, 25.2168) (-1.7962, 25.1661) (-1.7911, 25.1154) (-1.7856, 25.0647) (-1.7795, 25.014) (-1.7727, 24.9633) (-1.7652, 24.9126) (-1.7571, 24.8619) (-1.7484, 24.8111) (-1.7393, 24.7604) (-1.7297, 24.7097) (-1.7198, 24.659) (-1.7095, 24.6084) (-1.6988, 24.5577) (-1.6877, 24.507) (-1.6762, 24.4564) (-1.6642, 24.4057) (-1.6518, 24.3551) (-1.6391, 24.3045) (-1.6259, 24.2539) (-1.6124, 24.2034) (-1.5986, 24.1528) (-1.5844, 24.1023) (-1.5699, 24.0518) (-1.555, 24.0013) (-1.5398, 23.9509) (-1.5242, 23.9004) (-1.5083, 23.85) (-1.4921, 23.7996) (-1.4756, 23.7493) (-1.4587, 23.699) (-1.4415, 23.6487) (-1.424, 23.5984) (-1.4062, 23.5482) (-1.3881, 23.498) (-1.3697, 23.4478) (-1.351, 23.3976) (-1.3321, 23.3475) (-1.3128, 23.2975) (-1.2932, 23.2474) (-1.2733, 23.1974) (-1.2532, 23.1475) (-1.2327, 23.0975) (-1.212, 23.0477) (-1.191, 22.9978) (-1.1697, 22.948) (-1.1482, 22.8982) (-1.1264, 22.8485) (-1.1043, 22.7988) (-1.0819, 22.7491) (-1.0593, 22.6995) (-1.0364, 22.65) (-1.0133, 22.6005) (-0.9898, 22.551) (-0.9662, 22.5015) (-0.9422, 22.4522) (-0.9181, 22.4028) (-0.8936, 22.3535) (-0.8689, 22.3043) (-0.844, 22.2551) (-0.8188, 22.2059) (-0.7933, 22.1568) (-0.7676, 22.1078) (-0.7469, 22.0686) (-0.7312, 22.0392) (-0.7207, 22.0196) (-0.7155, 22.0098) knots 0 0 0 0 0 0 0.01428571 0.02857143 0.04285714 0.05714286 0.07142857 0.08571429 0.1 0.11428571 0.12857143 0.14285714 0.15714286 0.17142857 0.18571429 0.2 0.21428571 0.22857143 0.24285714 0.25714286 0.27142857 0.28571429 0.3 0.31428571 0.32857143 0.34285714 0.35714286 0.37142857 0.38571429 0.4 0.41428571 0.42857143 0.44285714 0.45714286 0.47142857 0.48571429 0.5 0.51428571 0.52857143 0.54285714 0.55714286 0.57142857 0.58571429 0.6 0.61428571 0.62857143 0.64285714 0.65714286 0.67142857 0.68571429 0.7 0.71428571 0.72857143 0.74285714 0.75714286 0.77142857 0.78571429 0.8 0.81428571 0.82857143 0.84285714 0.85714286 0.87142857 0.88571429 0.9 0.91428571 0.92857143 0.94285714 0.95714286 0.97142857 0.98571429 1 1 1 1 1 1
  arc A0 (-0.7155, 22.0098) -> (0.7155, 22.0098) centre (0, 48) ccw
  spline S1 degree 5 poles (0.7155, 22.0098) (0.7207, 22.0196) (0.7312, 22.0392) (0.7469, 22.0686) (0.7676, 22.1078) (0.7933, 22.1568) (0.8188, 22.2059) (0.844, 22.2551) (0.8689, 22.3043) (0.8936, 22.3535) (0.9181, 22.4028) (0.9422, 22.4522) (0.9662, 22.5015) (0.9898, 22.551) (1.0133, 22.6005) (1.0364, 22.65) (1.0593, 22.6995) (1.0819, 22.7491) (1.1043, 22.7988) (1.1264, 22.8485) (1.1482, 22.8982) (1.1697, 22.948) (1.191, 22.9978) (1.212, 23.0477) (1.2327, 23.0975) (1.2532, 23.1475) (1.2733, 23.1974) (1.2932, 23.2474) (1.3128, 23.2975) (1.3321, 23.3475) (1.351, 23.3976) (1.3697, 23.4478) (1.3881, 23.498) (1.4062, 23.5482) (1.424, 23.5984) (1.4415, 23.6487) (1.4587, 23.699) (1.4756, 23.7493) (1.4921, 23.7996) (1.5083, 23.85) (1.5242, 23.9004) (1.5398, 23.9509) (1.555, 24.0013) (1.5699, 24.0518) (1.5844, 24.1023) (1.5986, 24.1528) (1.6124, 24.2034) (1.6259, 24.2539) (1.6391, 24.3045) (1.6518, 24.3551) (1.6642, 24.4057) (1.6762, 24.4564) (1.6877, 24.507) (1.6988, 24.5577) (1.7095, 24.6084) (1.7198, 24.659) (1.7297, 24.7097) (1.7393, 24.7604) (1.7484, 24.8111) (1.7571, 24.8619) (1.7652, 24.9126) (1.7727, 24.9633) (1.7795, 25.014) (1.7856, 25.0647) (1.7911, 25.1154) (1.7962, 25.1661) (1.801, 25.2168) (1.8054, 25.2674) (1.8093, 25.3181) (1.8123, 25.3687) (1.814, 25.4192) (1.8137, 25.4596) (1.8124, 25.4899) (1.8111, 25.5101) (1.8102, 25.5201) knots -1 -1 -1 -1 -1 -1 -0.98571429 -0.97142857 -0.95714286 -0.94285714 -0.92857143 -0.91428571 -0.9 -0.88571429 -0.87142857 -0.85714286 -0.84285714 -0.82857143 -0.81428571 -0.8 -0.78571429 -0.77142857 -0.75714286 -0.74285714 -0.72857143 -0.71428571 -0.7 -0.68571429 -0.67142857 -0.65714286 -0.64285714 -0.62857143 -0.61428571 -0.6 -0.58571429 -0.57142857 -0.55714286 -0.54285714 -0.52857143 -0.51428571 -0.5 -0.48571429 -0.47142857 -0.45714286 -0.44285714 -0.42857143 -0.41428571 -0.4 -0.38571429 -0.37142857 -0.35714286 -0.34285714 -0.32857143 -0.31428571 -0.3 -0.28571429 -0.27142857 -0.25714286 -0.24285714 -0.22857143 -0.21428571 -0.2 -0.18571429 -0.17142857 -0.15714286 -0.14285714 -0.12857143 -0.11428571 -0.1 -0.08571429 -0.07142857 -0.05714286 -0.04285714 -0.02857143 -0.01428571 0 0 0 0 0 0
  line L1 (1.8102, 25.5201) -> (1.8082, 25.5465)
  arc A1 (2.6806, 26.6182) -> (1.8082, 25.5465) centre (2.805, 25.6259) ccw
  line L2 (2.6806, 26.6182) -> (-2.8127, 26.6352)
  arc A2 (-2.8127, 26.6352) -> (-2.6806, 26.6182) centre (0, 48) ccw
  arc A3 (-1.8082, 25.5465) -> (-2.6806, 26.6182) centre (-2.805, 25.6259) ccw
sketch "スケッチ3 (2)" plane through (0, 0, 12.7) normal (0, 0, 1) x (-1, 0, 0) in component "Rack"
  line L0 (61.0234, 25.3522) -> (61.0213, 25.3259)
  spline S0 degree 5 poles (61.0213, 25.3259) (61.0205, 25.3158) (61.0191, 25.2957) (61.0179, 25.2654) (61.0176, 25.225) (61.0192, 25.1745) (61.0222, 25.1239) (61.0262, 25.0732) (61.0306, 25.0226) (61.0353, 24.9719) (61.0404, 24.9212) (61.0459, 24.8705) (61.0521, 24.8198) (61.0589, 24.7691) (61.0663, 24.7183) (61.0745, 24.6676) (61.0831, 24.6169) (61.0923, 24.5662) (61.1018, 24.5155) (61.1117, 24.4648) (61.122, 24.4141) (61.1327, 24.3634) (61.1438, 24.3128) (61.1554, 24.2621) (61.1674, 24.2115) (61.1797, 24.1609) (61.1925, 24.1103) (61.2056, 24.0597) (61.2191, 24.0091) (61.233, 23.9586) (61.2471, 23.9081) (61.2617, 23.8576) (61.2766, 23.8071) (61.2918, 23.7566) (61.3073, 23.7062) (61.3232, 23.6558) (61.3395, 23.6054) (61.356, 23.5551) (61.3729, 23.5047) (61.39, 23.4544) (61.4075, 23.4042) (61.4253, 23.3539) (61.4434, 23.3037) (61.4618, 23.2536) (61.4805, 23.2034) (61.4995, 23.1533) (61.5188, 23.1032) (61.5384, 23.0532) (61.5582, 23.0032) (61.5784, 22.9532) (61.5988, 22.9033) (61.6195, 22.8534) (61.6405, 22.8036) (61.6618, 22.7538) (61.6834, 22.704) (61.7052, 22.6543) (61.7273, 22.6046) (61.7496, 22.5549) (61.7723, 22.5053) (61.7951, 22.4557) (61.8183, 22.4062) (61.8417, 22.3567) (61.8654, 22.3073) (61.8893, 22.2579) (61.9135, 22.2086) (61.9379, 22.1593) (61.9626, 22.11) (61.9876, 22.0609) (62.0128, 22.0117) (62.0382, 21.9626) (62.0639, 21.9136) (62.0847, 21.8744) (62.1003, 21.845) (62.1108, 21.8254) (62.1161, 21.8156) knots 0 0 0 0 0 0 0.01428571 0.02857143 0.04285714 0.05714286 0.07142857 0.08571429 0.1 0.11428571 0.12857143 0.14285714 0.15714286 0.17142857 0.18571429 0.2 0.21428571 0.22857143 0.24285714 0.25714286 0.27142857 0.28571429 0.3 0.31428571 0.32857143 0.34285714 0.35714286 0.37142857 0.38571429 0.4 0.41428571 0.42857143 0.44285714 0.45714286 0.47142857 0.48571429 0.5 0.51428571 0.52857143 0.54285714 0.55714286 0.57142857 0.58571429 0.6 0.61428571 0.62857143 0.64285714 0.65714286 0.67142857 0.68571429 0.7 0.71428571 0.72857143 0.74285714 0.75714286 0.77142857 0.78571429 0.8 0.81428571 0.82857143 0.84285714 0.85714286 0.87142857 0.88571429 0.9 0.91428571 0.92857143 0.94285714 0.95714286 0.97142857 0.98571429 1 1 1 1 1 1
  arc A0 (62.1161, 21.8156) -> (63.547, 21.8156) centre (62.8316, 47.8058) ccw
  spline S1 degree 5 poles (63.547, 21.8156) (63.5523, 21.8254) (63.5628, 21.845) (63.5784, 21.8744) (63.5992, 21.9136) (63.6249, 21.9626) (63.6503, 22.0117) (63.6755, 22.0609) (63.7005, 22.11) (63.7252, 22.1593) (63.7496, 22.2086) (63.7738, 22.2579) (63.7977, 22.3073) (63.8214, 22.3567) (63.8448, 22.4062) (63.868, 22.4557) (63.8909, 22.5053) (63.9135, 22.5549) (63.9358, 22.6046) (63.9579, 22.6543) (63.9797, 22.704) (64.0013, 22.7538) (64.0226, 22.8036) (64.0436, 22.8534) (64.0643, 22.9033) (64.0847, 22.9532) (64.1049, 23.0032) (64.1247, 23.0532) (64.1443, 23.1032) (64.1636, 23.1533) (64.1826, 23.2034) (64.2013, 23.2536) (64.2197, 23.3037) (64.2378, 23.3539) (64.2556, 23.4042) (64.2731, 23.4544) (64.2902, 23.5047) (64.3071, 23.5551) (64.3237, 23.6054) (64.3399, 23.6558) (64.3558, 23.7062) (64.3713, 23.7566) (64.3866, 23.8071) (64.4014, 23.8576) (64.416, 23.9081) (64.4301, 23.9586) (64.444, 24.0091) (64.4575, 24.0597) (64.4706, 24.1103) (64.4834, 24.1609) (64.4958, 24.2115) (64.5077, 24.2621) (64.5193, 24.3128) (64.5304, 24.3634) (64.5411, 24.4141) (64.5514, 24.4648) (64.5613, 24.5155) (64.5708, 24.5662) (64.58, 24.6169) (64.5886, 24.6676) (64.5968, 24.7183) (64.6043, 24.7691) (64.6111, 24.8198) (64.6172, 24.8705) (64.6227, 24.9212) (64.6278, 24.9719) (64.6325, 25.0226) (64.6369, 25.0732) (64.6409, 25.1239) (64.6439, 25.1745) (64.6455, 25.225) (64.6452, 25.2654) (64.644, 25.2957) (64.6426, 25.3158) (64.6418, 25.3259) knots -1 -1 -1 -1 -1 -1 -0.98571429 -0.97142857 -0.95714286 -0.94285714 -0.92857143 -0.91428571 -0.9 -0.88571429 -0.87142857 -0.85714286 -0.84285714 -0.82857143 -0.81428571 -0.8 -0.78571429 -0.77142857 -0.75714286 -0.74285714 -0.72857143 -0.71428571 -0.7 -0.68571429 -0.67142857 -0.65714286 -0.64285714 -0.62857143 -0.61428571 -0.6 -0.58571429 -0.57142857 -0.55714286 -0.54285714 -0.52857143 -0.51428571 -0.5 -0.48571429 -0.47142857 -0.45714286 -0.44285714 -0.42857143 -0.41428571 -0.4 -0.38571429 -0.37142857 -0.35714286 -0.34285714 -0.32857143 -0.31428571 -0.3 -0.28571429 -0.27142857 -0.25714286 -0.24285714 -0.22857143 -0.21428571 -0.2 -0.18571429 -0.17142857 -0.15714286 -0.14285714 -0.12857143 -0.11428571 -0.1 -0.08571429 -0.07142857 -0.05714286 -0.04285714 -0.02857143 -0.01428571 0 0 0 0 0 0
  line L1 (64.6418, 25.3259) -> (64.6397, 25.3522)
  arc A1 (65.5121, 26.4239) -> (64.6397, 25.3522) centre (65.6365, 25.4317) ccw
  line L2 (65.5121, 26.4239) -> (60.0188, 26.4409)
  arc A2 (60.0188, 26.4409) -> (60.151, 26.4239) centre (62.8316, 47.8058) ccw
  arc A3 (61.0234, 25.3522) -> (60.151, 26.4239) centre (60.0266, 25.4317) ccw
  line L3 (65.5121, 26.4239) -> (-65.5121, 26.8124)
  line L4 (-65.5121, 26.8124) -> (-65.5033, 29.8124)
  line L5 (-65.5033, 29.8124) -> (65.521, 29.4239)
  line L6 (65.521, 29.4239) -> (65.5121, 26.4239)
  point P0 (65.5121, 26.4239)
  point P1 (-65.5121, 26.8124)
  dimension "d19" = 3
  constraint perpendicular L3 L4
  constraint parallel L3 L5
  constraint parallel L4 L6
  constraint coincident P1 L3.end
  constraint coincident P0 A1.start
  measures "d19" distance of P0 L5.end
extrude "押し出し2'" add sketch "スケッチ3 (2)" against normal blind 12.7 contours L2 L3 L4 L5 L6 bodies 3 4 5 6 7 8 9 10 11 12 13 14 15 16 17 18 19 20 21 22 23 in component "Rack"
component "Spur Gear (24 teeth)" placed x (1, 0, 0) y (0, 1, 0) z (0, 0, 1) at (0, 0, 0)
component "Rack" placed x (1, 0, 0) y (0, 1, 0) z (0, 0, 1) at (0, 0, 0)
equation "d12 = ( ( 360 / 24 ) / 2 ) * 1 deg"
equation "d17 = ( ( 48 * PI ) / 24 ) * 1 mm"
